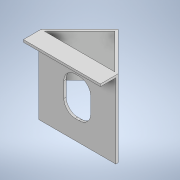
# Autodesk Inventor part: fixation_v02
Saved by Autodesk Inventor 2020 (Build 240168000, 168)
## iProperties
Created: 2021-04-13
Part Number: fixation_v02
Material: Generic
Document SubType Name: Modeling
Designer: KAMPFF-LAB-BEHAVIOR
Density: 1 g/cm^3
Appearance: Default
Author: KAMPFF-LAB-BEHAVIOR
Autodesk Inventor part; units mm, degrees
ref_plane "YZ Plane" through (0, 0, 0) normal (1, 0, 0) x (0, 1, 0)
ref_plane "XZ Plane" through (0, 0, 0) normal (0, 1, 0) x (-1, 0, 0)
ref_plane "XY Plane" through (0, 0, 0) normal (0, 0, 1) x (1, 0, 0)
sketch "Sketch1" plane through (0, 0, 0) normal (0, 0, 1) x (1, 0, 0)
  line L0 (-50, -50) -> (50, -50)
  line L1 (50, -50) -> (50, 50)
  line L2 (50, 50) -> (-50, 50)
  line L3 (-50, 50) -> (-50, -50)
  line L4 (-50, -50) -> (50, 50) construction
  line L5 (50, -50) -> (-50, 50) construction
  point P0 (0, 0)
  dimension "d0" = 100
  dimension "d1" = 100
  constraints: 12 end point, 2 midpoint, 2 parallel, 1 horizontal, 1 perpendicular
  measures "d0" distance of L2.end L1.end
  measures "d1" distance of L1.end L0.end
extrude "Extrusion1" add sketch "Sketch1" along normal blind 3
sketch "Sketch2" plane through (-50, 50, 0) normal (0, 1, 0) x (1, 0, 0)
  line L0 (0, 0) -> (100, 0) projected
  line L1 (0, 0) -> (50, 50)
  line L2 (50, 50) -> (52.1213, 47.8787)
  line L3 (52.1213, 47.8787) -> (2.1213, -2.1213)
  line L4 (2.1213, -2.1213) -> (0, 0)
  line L5 (0, 0) -> (70.7107, 0) construction
  line L6 (100, 0) -> (52.1213, 47.8787)
  line L7 (52.1213, 47.8787) -> (50, 45.7574)
  line L8 (50, 45.7574) -> (97.8787, -2.1213)
  line L9 (97.8787, -2.1213) -> (100, 0)
  point P0 (50, 0)
  dimension "d4" = 45
  dimension "d5" = 3
  dimension "d6" = 3
  constraints: 18 end point, 5 parallel, 2 perpendicular, 1 equal length, 1 horizontal, 1 point on line
  measures "d4" angle of L5 L1
  measures "d5" distance of L1.end L2.end
  measures "d6" distance of L7.end L2.end
extrude "Extrusion2" add sketch "Sketch2" against normal blind 55 contours L1 L2 L3 L0 | L0 L3 L4 | L8 L3 L6 L0 | L0 L9 L8
sketch "Sketch3" plane through (0, 0, 3) normal (0, 0, 1) x (1, 0, 0)
  line L0 (2.5, -25) -> (-2.5, -25)
  line L1 (-17.5, -10) -> (-17.5, 10)
  line L2 (-2.5, 25) -> (2.5, 25)
  line L3 (17.5, 10) -> (17.5, -10)
  line L4 (17.5, -25) -> (-17.5, 25) construction
  line L5 (-17.5, -25) -> (17.5, 25) construction
  arc A0 (-2.5, 25) -> (-17.5, 10) centre (-2.5, 10) ccw
  arc A1 (17.5, 10) -> (2.5, 25) centre (2.5, 10) ccw
  arc A2 (2.5, -25) -> (17.5, -10) centre (2.5, -10) ccw
  arc A3 (-17.5, -10) -> (-2.5, -25) centre (-2.5, -10) ccw
  point P0 (0, 0)
  dimension "d9" = 35
  dimension "d10" = 50
  dimension "d11" = 15
  constraints: 12 end point, 8 point on circle, 8 point on line, 8 tangent, 4 centre point, 3 equal radius, 2 midpoint, 2 parallel, 1 horizontal, 1 perpendicular
  measures "d9" distance of L4.end L5.end
  measures "d10" distance of L5.start L4.end
  measures "d11" radius of A0
extrude "Extrusion3" cut sketch "Sketch3" against normal blind 3
sketch "Sketch5" plane through (-50, 50, 3) normal (0, 1, 0) x (1, 0, 0)
  line L0 (0, 3) -> (0, 0) projected
  line L1 (0, 0) -> (100, 0)
  line L2 (100, 0) -> (100, -20)
  line L3 (100, -20) -> (0, -20)
  line L4 (0, -20) -> (0, 0)
  point P0 (50, 3)
  dimension "d16" = 100
  dimension "d17" = 20
  constraints: 8 end point, 2 parallel, 1 horizontal, 1 perpendicular
  measures "d16" distance of L2.end L3.end
  measures "d17" distance of L1.end L2.end
extrude "Extrusion5" add sketch "Sketch5" against normal blind 3
body "Solid1"
